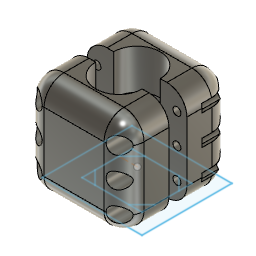
Tennis shaft connector (Autodesk Fusion 360 design; units mm, degrees)
Autodesk Fusion 360 part; units mm, degrees
sketch "Sketch1" plane through (0, 0, 0) normal (0, 0, 1) x (1, 0, 0)
  line L0 (-15, 20) -> (15, 20)
  line L1 (15, 20) -> (15, -5)
  line L2 (15, -5) -> (-15, -5)
  line L3 (-15, -5) -> (-15, 20)
  line L4 (-25, 30) -> (25, 30)
  line L5 (25, 30) -> (25, -15)
  line L6 (25, -15) -> (-25, -15)
  line L7 (-25, -15) -> (-25, 30)
  line L8 (8.504197, 20) -> (15, 13.510938)
  line L9 (8.513571, -5) -> (15, 1.484332)
  line L10 (-15, 1.500422) -> (-8.473728, -5)
  line L11 (-15, 13.506859) -> (-8.510889, 20)
  line L12 (-15, 13.506859) -> (-5.816055, 13.506859) construction
  dimension "d1" = 30
  dimension "d2" = 25
  dimension "d3" = 50
  dimension "d4" = 45
  dimension "d5" = 45.01779
  constraint horizontal L0
  constraint vertical L1
  constraint horizontal L2
  constraint vertical L3
  constraint horizontal L4
  constraint vertical L5
  constraint horizontal L6
  constraint vertical L7
  constraint horizontal L12
  measures "d1" distance of L0.start L0.end
  measures "d2" distance of L0.start L2.end
  measures "d3" distance of L4.start L4.end
  measures "d4" distance of L4.start L6.end
  measures "d5" angle of L11 L12
extrude "Extrude1" add sketch "Sketch1" along normal blind 50 contours L0 L3 L11 | L0 L1 L2 L3 L8 L9 L10 L11 | L0 L1 L8 | L2 L3 L10 | L1 L2 L9 | L4 L5 L6 L7 picked at (-12.836963, 17.83562) picked at (-2.826807, 11.666667) picked at (12.834732, 17.836979) picked at (-12.824576, -2.833193) picked at (12.837857, -2.838556) picked at (-2.824576, -11.666667) makes body 1
extrude "Extrude3" cut sketch "Sketch1" along normal blind 30 contours L0 L1 L2 L3 L8 L9 L10 L11 picked at (-2.826807, 11.666667) bodies 1
sketch "Sketch2" plane through (0, 0, 50) normal (0, 0, 1) x (-1, 0, 0)
  line L0 (25, 15) -> (-25, 15)
  line L1 (-25, 15) -> (-25, -30)
  line L2 (-25, -30) -> (25, -30)
  line L3 (25, -30) -> (25, 15)
  circle A0 centre (0, -7.5) radius 11.65
  dimension "d12" = 23.3
  measures "d12" diameter of A0
extrude "Extrude4" cut sketch "Sketch2" against normal blind 20 contours A0 picked at (-1.418741, -4.388763) bodies 1
sketch "Sketch3" plane through (0, -15, 0) normal (0, -1, 0) x (1, 0, 0)
  line L0 (-25, 0) -> (25, 0)
  line L1 (25, 0) -> (25, 50)
  line L2 (25, 50) -> (-25, 50)
  line L3 (-25, 50) -> (-25, 0)
  circle A0 centre (-20, 40.000001) radius 4
  circle A1 centre (-20, 40.000001) radius 2
  circle A2 centre (-20, 25.000001) radius 2
  circle A3 centre (-20, 25.000001) radius 4
  circle A4 centre (-20, 10.000001) radius 2
  circle A5 centre (-20, 10.000001) radius 4
  circle A6 centre (20, 40.000001) radius 2
  circle A7 centre (20, 40.000001) radius 4
  circle A8 centre (20, 25.000001) radius 2
  circle A9 centre (20, 25.000001) radius 4
  circle A10 centre (20, 10.000001) radius 4
  circle A11 centre (20, 10.000001) radius 2
  dimension "d15" = 8
  dimension "d16" = 4
  dimension "d17" = 8
  dimension "d18" = 4
  dimension "d19" = 8
  dimension "d20" = 4
  dimension "d21" = 8
  dimension "d22" = 4
  dimension "d23" = 8
  dimension "d24" = 4
  dimension "d25" = 8
  dimension "d26" = 4
  constraint concentric A0 A1
  constraint concentric A2 A3
  constraint concentric A4 A5
  constraint concentric A6 A7
  constraint concentric A8 A9
  constraint concentric A10 A11
  measures "d15" diameter of A0
  measures "d16" diameter of A1
  measures "d17" diameter of A3
  measures "d18" diameter of A2
  measures "d19" diameter of A5
  measures "d20" diameter of A4
  measures "d21" diameter of A7
  measures "d22" diameter of A6
  measures "d23" diameter of A9
  measures "d24" diameter of A8
  measures "d25" diameter of A10
  measures "d26" diameter of A11
extrude "Extrude5" cut sketch "Sketch3" against normal blind 45 contours A1 | A2 | A4 | A6 | A8 | A11 picked at (-19.734268, 39.083553) picked at (-20.614877, 24.900639) picked at (-20.614877, 9.900639) picked at (20.265732, 39.083553) picked at (19.385123, 24.900639) picked at (19.385123, 9.900639) bodies 1
extrude "Extrude7" cut sketch "Sketch3" against normal blind 15 contours A0 | A3 | A5 | A7 | A9 | A10 picked at (-16.689005, 39.701916) picked at (-16.689005, 24.701916) picked at (-16.681559, 9.801278) picked at (23.310995, 39.701916) picked at (23.310995, 24.701916) picked at (23.318441, 9.801278) bodies 1
sketch "Sketch4" plane through (0, 30, 0) normal (0, 1, 0) x (-1, 0, 0)
  circle A0 centre (-20, 25.000001) radius 2
  circle A1 centre (-20, 40.000001) radius 2
  circle A2 centre (-20, 10.000001) radius 2
  circle A3 centre (20, 25.000001) radius 2
  circle A4 centre (20, 40.000001) radius 2
  circle A5 centre (20, 10.000001) radius 2
  line L0 (-25, 0) -> (25, 0)
  line L1 (25, 0) -> (25, 50)
  line L2 (25, 50) -> (-25, 50)
  line L3 (-25, 50) -> (-25, 0)
  circle A6 centre (-20, 40.000001) radius 4
  circle A7 centre (-20, 25.000001) radius 4
  circle A8 centre (-20, 10.000001) radius 4
  circle A9 centre (20, 40.000001) radius 4
  circle A10 centre (20, 25.000001) radius 4
  circle A11 centre (20, 10.000001) radius 4
  dimension "d33" = 8
  dimension "d34" = 8
  dimension "d35" = 8
  dimension "d36" = 8
  dimension "d37" = 8
  dimension "d38" = 8
  constraint concentric A1 A6
  measures "d33" diameter of A6
  measures "d34" diameter of A7
  measures "d35" diameter of A8
  measures "d36" diameter of A9
  measures "d37" diameter of A10
  measures "d38" diameter of A11
extrude "Extrude8" cut sketch "Sketch4" against normal blind 15 contours A6 | A7 | A8 | A9 | A10 | A11 picked at (-16.689005, 39.701916) picked at (-16.689005, 24.701916) picked at (-16.681559, 9.801278) picked at (23.310995, 39.701916) picked at (23.310995, 24.701916) picked at (23.318441, 9.801278) bodies 1
fillet "Fillet4" radius 10 4 edges at (-25, -15, 25) (-25, 30, 25) (25, 30, 25) (25, -15, 25) on bodies 1
fillet "Fillet5" radius 10 8 edges at (-22.071068, 27.071068, 50) (-25, 7.5, 50) (-22.071068, -12.071068, 50) (0, -15, 50) (22.071068, -12.071068, 50) (25, 7.5, 50) (22.071068, 27.071068, 50) (0, 30, 50) on bodies 1
fillet "Fillet6" radius 10 8 edges at (22.071068, 27.071068, 0) (25, 7.5, 0) (22.071068, -12.071068, 0) (0, -15, 0) (-22.071068, -12.071068, 0) (-25, 7.5, 0) (-22.071068, 27.071068, 0) (0, 30, 0) on bodies 1
ref_plane "WorkPlane1" through (0, 7.5, 25) normal (0, 1, 0) x (-1, 0, 0)
split "Split1" by plane through (0, 7.5, 25) normal (0, 1, 0) bodies 1 makes body 2 at (-5, 30, 20)
move_body "Move1" bodies 1 to x (1, 0, 0) y (0, 1, 0) z (0, 0, 1) at (0, -9, 0)
sketch "Sketch5" plane through (25, 0, 0) normal (1, 0, 0) x (0, 1, 0)
  line L0 (-1.5, 10) -> (-1.5, 40)
  line L1 (-1.5, 40) -> (-14, 40)
  line L2 (-14, 40) -> (-14, 10)
  line L3 (-14, 10) -> (-1.5, 10)
  line L4 (30, 42.000001) -> (15, 42.000001)
  line L5 (15, 42.000001) -> (15, 38.000001)
  line L6 (15, 38.000001) -> (30, 38.000001)
  line L7 (30, 38.000001) -> (30, 42.000001)
  line L8 (15, 42.000001) -> (15, 38.000001)
  line L9 (30, 42.000001) -> (15, 42.000001)
  line L10 (30, 38.000001) -> (30, 42.000001)
  line L11 (15, 38.000001) -> (30, 38.000001)
  line L12 (15, 27.000001) -> (15, 23.000001)
  line L13 (30, 27.000001) -> (15, 27.000001)
  line L14 (30, 23.000001) -> (30, 27.000001)
  line L15 (15, 23.000001) -> (30, 23.000001)
  line L16 (15, 12.000001) -> (15, 8.000001)
  line L17 (30, 12.000001) -> (15, 12.000001)
  line L18 (30, 8.000001) -> (30, 12.000001)
  line L19 (15, 8.000001) -> (30, 8.000001)
  dimension "d47" = 15
  dimension "d48" = 4
  dimension "d49" = 15
  dimension "d50" = 4
  dimension "d51" = 15
  dimension "d52" = 4
  dimension "d53" = 15
  dimension "d54" = 4
  constraint horizontal L4
  constraint vertical L5
  constraint horizontal L6
  constraint vertical L7
  constraint horizontal L9
  constraint vertical L8
  constraint horizontal L11
  constraint vertical L10
  constraint horizontal L13
  constraint vertical L12
  constraint horizontal L15
  constraint vertical L14
  constraint horizontal L17
  constraint vertical L16
  constraint horizontal L19
  constraint vertical L18
sketch "Sketch6" plane through (-25, 0, 0) normal (-1, 0, 0) x (0, -1, 0)
  line L0 (-7.5, 10) -> (-7.5, 40)
  line L1 (-7.5, 40) -> (-20, 40)
  line L2 (-20, 40) -> (-20, 10)
  line L3 (-20, 10) -> (-7.5, 10)
  line L4 (-30, 42.000001) -> (-15, 42.000001)
  line L5 (-15, 42.000001) -> (-15, 38.000001)
  line L6 (-15, 38.000001) -> (-30, 38.000001)
  line L7 (-30, 38.000001) -> (-30, 42.000001)
  line L8 (-30, 27.000001) -> (-15, 27.000001)
  line L9 (-30, 23.000001) -> (-30, 27.000001)
  line L10 (-15, 23.000001) -> (-30, 23.000001)
  line L11 (-15, 27.000001) -> (-15, 23.000001)
  line L12 (-30, 12.000001) -> (-15, 12.000001)
  line L13 (-30, 8.000001) -> (-30, 12.000001)
  line L14 (-15, 8.000001) -> (-30, 8.000001)
  line L15 (-15, 12.000001) -> (-15, 8.000001)
  dimension "d55" = 15
  dimension "d56" = 15
  dimension "d57" = 15
  constraint horizontal L4
  constraint vertical L5
  constraint horizontal L6
  constraint vertical L7
  constraint horizontal L8
  constraint vertical L11
  constraint horizontal L10
  constraint vertical L9
  constraint horizontal L12
  constraint vertical L15
  constraint horizontal L14
  constraint vertical L13
extrude "Extrude9" cut sketch "Sketch6" against normal blind 2 contours L2 L3 L12 L13 L14 L15 | L2 L3 L12 L15 | L1 L2 L5 L6 | L1 L2 L4 L5 L6 L7 | L2 L8 L9 L10 | L2 L8 L10 L11 picked at (-26.666667, 10) picked at (-16.666667, 10.666667) picked at (-18.333333, 39.333334) picked at (-26.666667, 40) picked at (-23.333333, 24.333334) picked at (-18.333333, 25.666667) bodies 2
extrude "Extrude10" cut sketch "Sketch5" against normal blind 2 contours L4 L5 L6 L7 L8 L9 L10 L11 | L12 L13 L14 L15 | L16 L17 L18 L19 picked at (20, 40.666667) picked at (20, 25.666667) picked at (20, 10.666667) bodies 2
